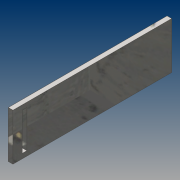
# Autodesk Inventor part: 02_Tam_hong
Saved by Autodesk Inventor 2021 (Build 250183000, 183)
## iProperties
Created: 2024-04-07
Part Number: 02_Tam_hong
Material: Stainless Steel, Austenitic
Document SubType Name: Modeling
Designer: Admin
Density: 8 g/cm^3
Appearance: Semi-Polished
Mass: 2560 g
Surface Area: 724 cm^2
Volume: 320 cm^3
Author: Admin
Autodesk Inventor part; units mm, degrees
ref_plane "YZ Plane" through (0, 0, 0) normal (1, 0, 0) x (0, 1, 0)
ref_plane "XZ Plane" through (0, 0, 0) normal (0, 1, 0) x (-1, 0, 0)
ref_plane "XY Plane" through (0, 0, 0) normal (0, 0, 1) x (1, 0, 0)
sketch "Sketch1" plane through (0, 0, 0) normal (1, 0, 0) x (0, 1, 0)
  line L0 (-50, 160) -> (50, 160)
  line L1 (50, 160) -> (50, -160)
  line L2 (50, -160) -> (-50, -160)
  line L3 (-50, -160) -> (-50, 160)
  line L4 (-50, 160) -> (50, -160) construction
  line L5 (50, 160) -> (-50, -160) construction
  point P0 (0, 0)
  dimension "d0" = 320
  dimension "d1" = 100
  constraints: 12 end point, 2 midpoint, 2 parallel, 1 horizontal, 1 perpendicular
  measures "d0" distance of L0.end L1.end
  measures "d1" distance of L1.end L2.end
extrude "Extrusion1" add sketch "Sketch1" along normal blind 10
sketch "Sketch2" plane through (0, 0, 0) normal (-1, 0, 0) x (0, 0, 1)
  line L0 (-160, -50) -> (-160, 50) projected
  line L1 (160, -50) -> (-160, -50) projected
  line L2 (160, 50) -> (160, -50) projected
  line L3 (-160, 50) -> (160, 50) projected
  line L4 (180, 50) -> (-180, 50)
  line L5 (-180, 50) -> (-180, -50)
  line L6 (-180, -50) -> (180, -50)
  line L7 (180, -50) -> (180, 50)
  line L8 (180, 50) -> (-180, -50) construction
  line L9 (-180, 50) -> (180, -50) construction
  line L10 (150, 30) -> (170, 30)
  line L11 (170, 30) -> (170, -30)
  line L12 (170, -30) -> (150, -30)
  line L13 (150, -30) -> (150, 30)
  line L14 (160, 50) -> (160, -50) projected
  line L15 (150, 30) -> (170, -30) construction
  line L16 (170, 30) -> (150, -30) construction
  point P0 (0, 0)
  point P1 (160, 0)
  point P2 (160, 30)
  point P3 (160, -30)
  dimension "d4" = 20
  dimension "d5" = 10
  dimension "d6" = 60
  constraints: 24 end point, 5 midpoint, 4 parallel, 2 horizontal, 2 perpendicular, 1 horizontal alignment
  measures "d4" distance between parallel lines of L0 L5
  measures "d5" distance between parallel lines of L2 L11
  measures "d6" distance between parallel lines of L10 L12
extrude "Extrusion2" add sketch "Sketch2" against normal blind 10 contours L2 L12 L11 L10 L4 L7 L6 | L2 L10 L11 L12
extrude "Extrusion3" cut sketch "Sketch2" against normal blind 36.25 contours L12 L13 L10 L2
mirror "Mirror1" about plane through (0, 0, 0) normal (0, 0, 1) of "Extrusion3", "Extrusion2"
chamfer "Chamfer1" distance 16.5 angle 45 1 edges at (5, 50, 180)
body "Solid1"
